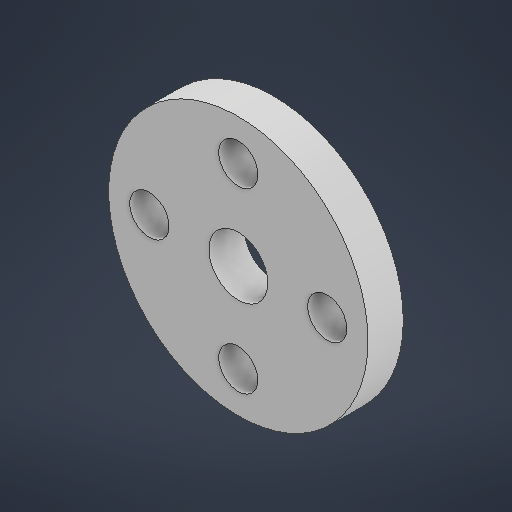
# Autodesk Inventor part: проставка для колеса
Saved by Autodesk Inventor 2025 (Build 290162000, 162)
## iProperties
Created: 2025-10-15
Part Number: проставка для колеса
Material: Типовые
Document SubType Name: Modeling
Designer: Phantom
Density: 1 g/cm^3
Appearance: По умолчанию
Author: Phantom
Autodesk Inventor part; units mm, degrees
ref_plane "YZ Plane" through (0, 0, 0) normal (1, 0, 0) x (0, 1, 0)
ref_plane "XZ Plane" through (0, 0, 0) normal (0, 1, 0) x (-1, 0, 0)
ref_plane "XY Plane" through (0, 0, 0) normal (0, 0, 1) x (1, 0, 0)
sketch "Эскиз1" plane through (0, 0, 0) normal (0, 0, 1) x (1, 0, 0)
  circle A0 centre (0, 0) radius 16.5
  circle A1 centre (0, 0) radius 3.75
  circle A2 centre (0, 0) radius 11.32
  circle A3 centre (-11.32, 0) radius 2.5
  circle A4 centre (0, -11.32) radius 2.5
  circle A5 centre (11.32, 0) radius 2.5
  circle A6 centre (0, 11.32) radius 2.5
  dimension "d2" = 22.64
  dimension "d0" = 33
  dimension "d1" = 7.5
  dimension "d3" = 5
  dimension "d6" = 360
  constraints: 6 centre point, 3 coincident, 1 horizontal alignment, 11 other
  measures "d0" diameter of A0
  measures "d1" diameter of A1
  measures "d3" diameter of A3
extrude "Выдавливание1" add sketch "Эскиз1" along normal blind 4.5 contours A0 | A5 A2 A4 A3 A6
